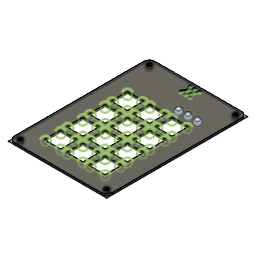
Macropad (Autodesk Fusion 360 archive; units mm, degrees)
design "Macropad Top"
part number: 2026-01-12-19-00-30-653
Autodesk Fusion 360 part; units mm, degrees
sketch "plate-2026-01-11T15_22_50.365Z" plane through (0, 0, 0) normal (0, 0, 1) x (1, 0, 0)
  line L0 (3.025, -2.525) -> (16.025, -2.525)
  line L1 (3.025, -16.525) -> (16.025, -16.525)
  line L2 (2.525, -3.025) -> (2.525, -16.025)
  line L3 (16.525, -3.025) -> (16.525, -16.025)
  arc A0 (3.025, -2.525) -> (2.525, -3.025) centre (3.025, -3.025) ccw
  arc A1 (16.525, -3.025) -> (16.025, -2.525) centre (16.025, -3.025) ccw
  arc A2 (2.525, -16.025) -> (3.025, -16.525) centre (3.025, -16.025) ccw
  arc A3 (16.025, -16.525) -> (16.525, -16.025) centre (16.025, -16.025) ccw
  line L4 (22.075, -2.525) -> (35.075, -2.525)
  line L5 (22.075, -16.525) -> (35.075, -16.525)
  line L6 (21.575, -3.025) -> (21.575, -16.025)
  line L7 (35.575, -3.025) -> (35.575, -16.025)
  arc A4 (22.075, -2.525) -> (21.575, -3.025) centre (22.075, -3.025) ccw
  arc A5 (35.575, -3.025) -> (35.075, -2.525) centre (35.075, -3.025) ccw
  arc A6 (21.575, -16.025) -> (22.075, -16.525) centre (22.075, -16.025) ccw
  arc A7 (35.075, -16.525) -> (35.575, -16.025) centre (35.075, -16.025) ccw
  line L8 (41.125, -2.525) -> (54.125, -2.525)
  line L9 (41.125, -16.525) -> (54.125, -16.525)
  line L10 (40.625, -3.025) -> (40.625, -16.025)
  line L11 (54.625, -3.025) -> (54.625, -16.025)
  arc A8 (41.125, -2.525) -> (40.625, -3.025) centre (41.125, -3.025) ccw
  arc A9 (54.625, -3.025) -> (54.125, -2.525) centre (54.125, -3.025) ccw
  arc A10 (40.625, -16.025) -> (41.125, -16.525) centre (41.125, -16.025) ccw
  arc A11 (54.125, -16.525) -> (54.625, -16.025) centre (54.125, -16.025) ccw
  line L12 (3.025, -21.575) -> (16.025, -21.575)
  line L13 (3.025, -35.575) -> (16.025, -35.575)
  line L14 (2.525, -22.075) -> (2.525, -35.075)
  line L15 (16.525, -22.075) -> (16.525, -35.075)
  arc A12 (3.025, -21.575) -> (2.525, -22.075) centre (3.025, -22.075) ccw
  arc A13 (16.525, -22.075) -> (16.025, -21.575) centre (16.025, -22.075) ccw
  arc A14 (2.525, -35.075) -> (3.025, -35.575) centre (3.025, -35.075) ccw
  arc A15 (16.025, -35.575) -> (16.525, -35.075) centre (16.025, -35.075) ccw
  line L16 (22.075, -21.575) -> (35.075, -21.575)
  line L17 (22.075, -35.575) -> (35.075, -35.575)
  line L18 (21.575, -22.075) -> (21.575, -35.075)
  line L19 (35.575, -22.075) -> (35.575, -35.075)
  arc A16 (22.075, -21.575) -> (21.575, -22.075) centre (22.075, -22.075) ccw
  arc A17 (35.575, -22.075) -> (35.075, -21.575) centre (35.075, -22.075) ccw
  arc A18 (21.575, -35.075) -> (22.075, -35.575) centre (22.075, -35.075) ccw
  arc A19 (35.075, -35.575) -> (35.575, -35.075) centre (35.075, -35.075) ccw
  line L20 (41.125, -21.575) -> (54.125, -21.575)
  line L21 (41.125, -35.575) -> (54.125, -35.575)
  line L22 (40.625, -22.075) -> (40.625, -35.075)
  line L23 (54.625, -22.075) -> (54.625, -35.075)
  arc A20 (41.125, -21.575) -> (40.625, -22.075) centre (41.125, -22.075) ccw
  arc A21 (54.625, -22.075) -> (54.125, -21.575) centre (54.125, -22.075) ccw
  arc A22 (40.625, -35.075) -> (41.125, -35.575) centre (41.125, -35.075) ccw
  arc A23 (54.125, -35.575) -> (54.625, -35.075) centre (54.125, -35.075) ccw
  line L24 (3.025, -40.625) -> (16.025, -40.625)
  line L25 (3.025, -54.625) -> (16.025, -54.625)
  line L26 (2.525, -41.125) -> (2.525, -54.125)
  line L27 (16.525, -41.125) -> (16.525, -54.125)
  arc A24 (3.025, -40.625) -> (2.525, -41.125) centre (3.025, -41.125) ccw
  arc A25 (16.525, -41.125) -> (16.025, -40.625) centre (16.025, -41.125) ccw
  arc A26 (2.525, -54.125) -> (3.025, -54.625) centre (3.025, -54.125) ccw
  arc A27 (16.025, -54.625) -> (16.525, -54.125) centre (16.025, -54.125) ccw
  line L28 (22.075, -40.625) -> (35.075, -40.625)
  line L29 (22.075, -54.625) -> (35.075, -54.625)
  line L30 (21.575, -41.125) -> (21.575, -54.125)
  line L31 (35.575, -41.125) -> (35.575, -54.125)
  arc A28 (22.075, -40.625) -> (21.575, -41.125) centre (22.075, -41.125) ccw
  arc A29 (35.575, -41.125) -> (35.075, -40.625) centre (35.075, -41.125) ccw
  arc A30 (21.575, -54.125) -> (22.075, -54.625) centre (22.075, -54.125) ccw
  arc A31 (35.075, -54.625) -> (35.575, -54.125) centre (35.075, -54.125) ccw
  line L32 (41.125, -40.625) -> (54.125, -40.625)
  line L33 (41.125, -54.625) -> (54.125, -54.625)
  line L34 (40.625, -41.125) -> (40.625, -54.125)
  line L35 (54.625, -41.125) -> (54.625, -54.125)
  arc A32 (41.125, -40.625) -> (40.625, -41.125) centre (41.125, -41.125) ccw
  arc A33 (54.625, -41.125) -> (54.125, -40.625) centre (54.125, -41.125) ccw
  arc A34 (40.625, -54.125) -> (41.125, -54.625) centre (41.125, -54.125) ccw
  arc A35 (54.125, -54.625) -> (54.625, -54.125) centre (54.125, -54.125) ccw
  line L36 (3.025, -59.675) -> (16.025, -59.675)
  line L37 (3.025, -73.675) -> (16.025, -73.675)
  line L38 (2.525, -60.175) -> (2.525, -73.175)
  line L39 (16.525, -60.175) -> (16.525, -73.175)
  arc A36 (3.025, -59.675) -> (2.525, -60.175) centre (3.025, -60.175) ccw
  arc A37 (16.525, -60.175) -> (16.025, -59.675) centre (16.025, -60.175) ccw
  arc A38 (2.525, -73.175) -> (3.025, -73.675) centre (3.025, -73.175) ccw
  arc A39 (16.025, -73.675) -> (16.525, -73.175) centre (16.025, -73.175) ccw
  line L40 (22.075, -59.675) -> (35.075, -59.675)
  line L41 (22.075, -73.675) -> (35.075, -73.675)
  line L42 (21.575, -60.175) -> (21.575, -73.175)
  line L43 (35.575, -60.175) -> (35.575, -73.175)
  arc A40 (22.075, -59.675) -> (21.575, -60.175) centre (22.075, -60.175) ccw
  arc A41 (35.575, -60.175) -> (35.075, -59.675) centre (35.075, -60.175) ccw
  arc A42 (21.575, -73.175) -> (22.075, -73.675) centre (22.075, -73.175) ccw
  arc A43 (35.075, -73.675) -> (35.575, -73.175) centre (35.075, -73.175) ccw
  line L44 (41.125, -59.675) -> (54.125, -59.675)
  line L45 (41.125, -73.675) -> (54.125, -73.675)
  line L46 (40.625, -60.175) -> (40.625, -73.175)
  line L47 (54.625, -60.175) -> (54.625, -73.175)
  arc A44 (41.125, -59.675) -> (40.625, -60.175) centre (41.125, -60.175) ccw
  arc A45 (54.625, -60.175) -> (54.125, -59.675) centre (54.125, -60.175) ccw
  arc A46 (40.625, -73.175) -> (41.125, -73.675) centre (41.125, -73.175) ccw
  arc A47 (54.125, -73.675) -> (54.625, -73.175) centre (54.125, -73.175) ccw
  line L48 (-12.953, 31.685) -> (71.047, 31.685)
  line L49 (71.047, 31.685) -> (71.047, -88.815)
  line L50 (71.047, -88.815) -> (-12.953, -88.815)
  line L51 (-12.953, -88.815) -> (-12.953, 31.685)
  circle A48 centre (-7.953, 26.685) radius 1.7
  circle A49 centre (66.047, 26.685) radius 1.7
  circle A50 centre (-7.953, -83.815) radius 1.7
  circle A51 centre (66.047, -83.815) radius 1.7
  circle A52 centre (45.395, 6.3907) radius 1.75
  circle A53 centre (53.395, 6.5335) radius 1.75
  circle A54 centre (37.395, 6.3572) radius 1.75
  line L52 (33.7164, 21.1039) -> (31.6922, 24.7112)
  line L53 (31.6922, 24.7112) -> (33.7164, 28.3186)
  line L54 (33.7164, 28.3186) -> (33.7164, 29.3696)
  line L55 (33.7164, 29.3696) -> (32.4295, 29.3696)
  line L56 (32.4295, 29.3696) -> (32.4295, 28.3186)
  line L57 (32.4295, 28.3186) -> (31.089, 25.7088)
  line L58 (31.089, 25.7088) -> (31.0622, 25.7088)
  line L59 (31.0622, 25.7088) -> (29.7082, 29.3696)
  line L60 (29.7082, 29.3696) -> (28.3945, 29.3696)
  line L61 (28.3945, 29.3696) -> (27.0272, 25.7088)
  line L62 (27.0272, 25.7088) -> (27.0004, 25.7088)
  line L63 (27.0004, 25.7088) -> (25.5794, 28.3186)
  line L64 (25.5794, 28.3186) -> (25.5794, 29.3696)
  line L65 (25.5794, 29.3696) -> (24.3997, 29.3696)
  line L66 (24.3997, 29.3696) -> (24.3997, 28.3186)
  line L67 (24.3997, 28.3186) -> (26.4373, 24.7112)
  line L68 (26.4373, 24.7112) -> (24.3997, 21.1039)
  line L69 (24.3997, 21.1039) -> (24.3997, 20.0529)
  line L70 (24.3997, 20.0529) -> (25.5794, 20.0529)
  line L71 (25.5794, 20.0529) -> (25.5794, 21.1039)
  line L72 (25.5794, 21.1039) -> (27.0004, 23.7137)
  line L73 (27.0004, 23.7137) -> (27.0272, 23.7137)
  line L74 (27.0272, 23.7137) -> (28.3945, 20.0529)
  line L75 (28.3945, 20.0529) -> (29.7082, 20.0529)
  line L76 (29.7082, 20.0529) -> (31.0622, 23.7137)
  line L77 (31.0622, 23.7137) -> (31.089, 23.7137)
  line L78 (31.089, 23.7137) -> (32.4295, 21.1039)
  line L79 (32.4295, 21.1039) -> (32.4295, 20.0529)
  line L80 (32.4295, 20.0529) -> (33.7164, 20.0529)
  line L81 (33.7164, 20.0529) -> (33.7164, 21.1039)
  line L82 (30.4723, 24.7112) -> (29.105, 21.1039)
  line L83 (29.105, 21.1039) -> (29.0782, 21.1039)
  line L84 (29.0782, 21.1039) -> (27.6572, 24.7112)
  line L85 (27.6572, 24.7112) -> (29.0782, 28.3186)
  line L86 (29.0782, 28.3186) -> (29.105, 28.3186)
  line L87 (29.105, 28.3186) -> (30.4723, 24.7112)
  dimension "d1" = 84
  dimension "d2" = 120.5
  dimension "d3" = 15.14
  dimension "d4" = 15.478
  dimension "d5" = 3.4
  dimension "d6" = 5
  dimension "d7" = 5
  dimension "d8" = 3.4
  dimension "d9" = 5
  dimension "d10" = 5
  dimension "d11" = 3.4
  dimension "d12" = 5
  dimension "d13" = 5
  dimension "d14" = 3.4
  dimension "d15" = 5
  dimension "d16" = 5
  dimension "d17" = 3.5
  dimension "d18" = 3.5
  dimension "d19" = 3.5
  dimension "d20" = 17.652
  dimension "d21" = 8
  dimension "d22" = 8
  constraint horizontal L48
  constraint vertical L49
  constraint horizontal L50
  constraint vertical L51
  measures "d1" distance of L48.start L48.end
  measures "d2" distance of L48.start L50.end
  measures "d3" distance of L37 L50
  measures "d4" distance of L38 L51
  measures "d5" diameter of A48
  measures "d6" distance of L48 A48.centre
  measures "d7" distance of L51 A48.centre
  measures "d8" diameter of A49
  measures "d9" distance of L48 A49.centre
  measures "d10" distance of L49 A49.centre
  measures "d11" diameter of A50
  measures "d12" distance of L51 A50.centre
  measures "d13" distance of L50 A50.centre
  measures "d14" diameter of A51
  measures "d15" distance of L49 A51.centre
  measures "d16" distance of L50 A51.centre
  measures "d17" diameter of A52
  measures "d18" diameter of A53
  measures "d19" diameter of A54
  measures "d20" distance of L49 A53.centre
  measures "d21" horizontal distance of A52.centre A53.centre
  measures "d22" horizontal distance of A52.centre A54.centre
extrude "Extrude1" add sketch "plate-2026-01-11T15_22_50.365Z" along normal blind 1.5 contours L48 L49 L50 L51 | L52 L53 L54 L55 L56 L57 L58 L59 L60 L61 L62 L63 L64 L65 L66 L67 L68 L69 L70 L71 L72 L73 L74 L75 L76 L77 L78 L79 L80 L81 | L82 L83 L84 L85 L86 L87
fillet "Fillet1" radius 5 1 edges at (71.047, -88.815, 0.75)
fillet "Fillet2" radius 5 1 edges at (-12.953, -88.815, 0.75)
fillet "Fillet3" radius 5 1 edges at (-12.953, 31.685, 0.75)
fillet "Fillet4" radius 5 1 edges at (71.047, 31.685, 0.75)
move_body "Move1" bodies 1 to x (1, 0, 0) y (0, 1, 0) z (0, 0, 1) at (0, 0, -1.5)
extrude "Extrude2" cut sketch "plate-2026-01-11T15_22_50.365Z" against normal blind 0.5 contours L52 L53 L54 L55 L56 L57 L58 L59 L60 L61 L62 L63 L64 L65 L66 L67 L68 L69 L70 L71 L72 L73 L74 L75 L76 L77 L78 L79 L80 L81
move_body "Move2" bodies 1 to x (1, 0, 0) y (0, 1, 0) z (0, 0, 1) at (0, 0, 1.5)
equation "d3 = 5.14 mm + 10 mm"
equation "d4 = 5.478 mm + 10 mm"
equation "d20 = 7.652 mm + 10 mm"
